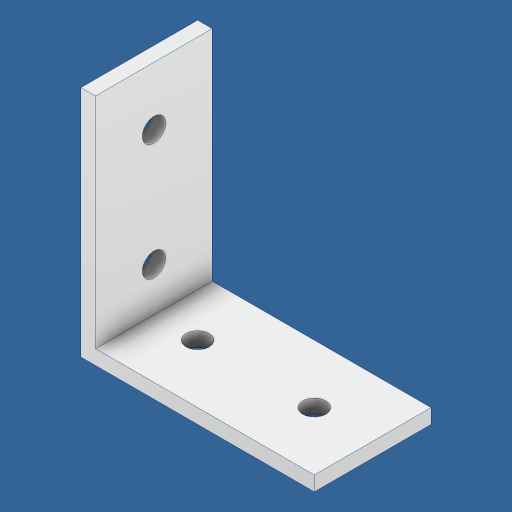
# Autodesk Inventor part: Centerpiece-90CornerBracket
Saved by Autodesk Inventor 2023 (Build 270158030, 158C)
## iProperties
Created: 2022-11-01
Part Number: Centerpiece-90CornerBracket
Material: Aluminum 6061-AHC
Document SubType Name: Modeling
Designer: Nebil
Density: 2.7 g/cm^3
Appearance: Aluminum - Flat
Mass: 20.7362 g
Surface Area: 58.2682 cm^2
Volume: 7.68008 cm^3
Author: Nebil
Autodesk Inventor part; units mm, degrees
ref_plane "YZ Plane" through (0, 0, 0) normal (1, 0, 0) x (0, 1, 0)
ref_plane "XZ Plane" through (0, 0, 0) normal (0, 1, 0) x (-1, 0, 0)
ref_plane "XY Plane" through (0, 0, 0) normal (0, 0, 1) x (1, 0, 0)
sketch "Sketch1" plane through (0, 0, 0) normal (0, 0, 1) x (1, 0, 0)
  line L0 (0, 0) -> (0, 50.8)
  line L1 (0, 50.8) -> (3.175, 50.8)
  line L2 (3.175, 50.8) -> (3.175, 3.175)
  line L3 (3.175, 3.175) -> (50.8, 3.175)
  line L4 (0, 0) -> (50.8, 0)
  line L5 (50.8, 3.175) -> (50.8, 0)
  dimension "d0" = 50.8
  dimension "d1" = 3.175
  dimension "d2" = 47.625
  dimension "d5" = 50.8
  dimension "d6" = 3.175
  constraints: 12 end point, 3 vertical, 2 perpendicular
  measures "d0" distance of L0.start L0.end
  measures "d1" distance of L0.end L1.end
  measures "d2" distance of L1.end L2.end
  measures "d5" distance of L0.start L4.end
  measures "d6" distance of L3.end L4.end
extrude "Extrusion1" add sketch "Sketch1" along normal blind 25.4
sketch "Sketch2" plane through (3.175, 3.175, 0) normal (1, 0, 0) x (0, 0, -1)
  line L0 (0, 47.625) -> (-25.4, 47.625) projected
  line L1 (-25.4, 0) -> (-25.4, 47.625) projected
  line L2 (0, 0) -> (-25.4, 0) projected
  point P0 (0, -3.175)
  point P1 (-12.7, 34.925)
  point P2 (-12.7, 9.525)
  dimension "d16" = 12.7
  dimension "d17" = 12.7
  dimension "d19" = 12.7
  dimension "d34" = 25.4
  measures "d16" distance from line of L0 point (-12.7, 34.925)
  measures "d17" distance from line of L1 point (-12.7, 34.925)
  measures "d19" distance from line of L1 point (-12.7, 9.525)
  measures "d34" distance of point (-12.7, 9.525) point (-12.7, 34.925)
hole "Hole1" at (3.175, 38.1, 12.7) at (3.175, 12.7, 12.7) direction (-1, 0, 0) diameter 5.08 end through all
sketch "Sketch3" plane through (3.175, 3.175, 0) normal (0, 1, 0) x (1, 0, 0)
  line L0 (47.625, -25.4) -> (0, -25.4) projected
  line L1 (0, 0) -> (0, -25.4) projected
  line L2 (47.625, 0) -> (47.625, -25.4) projected
  point P0 (-3.175, 0)
  point P1 (9.525, -12.7)
  point P2 (34.925, -12.7)
  dimension "d23" = 12.7
  dimension "d25" = 12.7
  dimension "d26" = 12.7
  dimension "d35" = 25.4
  measures "d23" distance from line of L0 point (9.525, -12.7)
  measures "d25" distance from line of L2 point (34.925, -12.7)
  measures "d26" distance from line of L0 point (34.925, -12.7)
  measures "d35" distance of point (34.925, -12.7) point (9.525, -12.7)
hole "Hole2" at (12.7, 3.175, 12.7) at (38.1, 3.175, 12.7) direction (0, -1, 0) diameter 5.08 end through all
equation "\"d2\" = d0 - d6"
equation "\"d6\" = d1"
body "Solid1"
